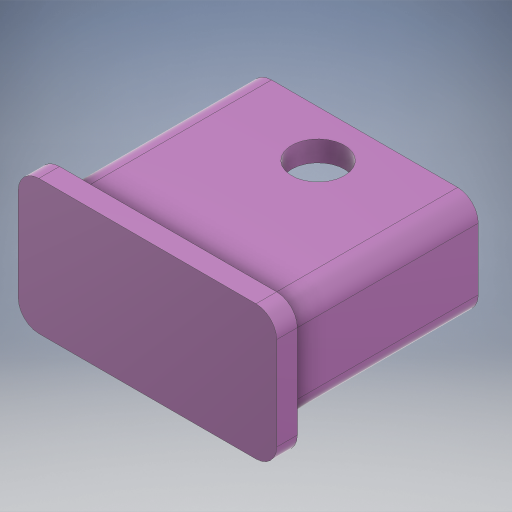
# Autodesk Inventor part: Короб подшипника
Saved by Autodesk Inventor 2023 (Build 270158000, 158)
## iProperties
Created: 2022-10-30
Part Number: Короб подшипника
Material: Типовые
Document SubType Name: Modeling
Designer: Admin
Density: 1 g/cm^3
Appearance: По умолчанию
Author: Admin
Autodesk Inventor part; units mm, degrees
ref_plane "YZ Plane" through (0, 0, 0) normal (1, 0, 0) x (0, 1, 0)
ref_plane "XZ Plane" through (0, 0, 0) normal (0, 1, 0) x (-1, 0, 0)
ref_plane "XY Plane" through (0, 0, 0) normal (0, 0, 1) x (1, 0, 0)
sketch "Эскиз1" plane through (0, 0, 0) normal (0, 0, 1) x (1, 0, 0)
  line L0 (-10.5, -6.5) -> (10.5, -6.5)
  line L1 (12.5, -4.5) -> (12.5, 4.5)
  line L2 (10.5, 6.5) -> (-10.5, 6.5)
  line L3 (-12.5, 4.5) -> (-12.5, -4.5)
  line L4 (-12.5, -6.5) -> (12.5, 6.5) construction
  line L5 (12.5, -6.5) -> (-12.5, 6.5) construction
  line L6 (-9, 5) -> (9, 5)
  line L7 (11, 3) -> (11, -3)
  line L8 (9, -5) -> (-9, -5)
  line L9 (-11, -3) -> (-11, 3)
  arc A0 (-10.5, 6.5) -> (-12.5, 4.5) centre (-10.5, 4.5) ccw
  arc A1 (12.5, 4.5) -> (10.5, 6.5) centre (10.5, 4.5) ccw
  arc A2 (10.5, -6.5) -> (12.5, -4.5) centre (10.5, -4.5) ccw
  arc A3 (-12.5, -4.5) -> (-10.5, -6.5) centre (-10.5, -4.5) ccw
  arc A4 (-9, 5) -> (-11, 3) centre (-9, 3) ccw
  arc A5 (11, 3) -> (9, 5) centre (9, 3) ccw
  arc A6 (9, -5) -> (11, -3) centre (9, -3) ccw
  arc A7 (-11, -3) -> (-9, -5) centre (-9, -3) ccw
  line L10 (-9, 3) -> (9, 3)
  line L11 (9, 3) -> (9, -3)
  line L12 (9, -3) -> (-9, -3)
  line L13 (-9, -3) -> (-9, 3)
  line L14 (-9, 3) -> (9, -3) construction
  line L15 (9, 3) -> (-9, -3) construction
  point P0 (0, 0)
  dimension "d0" = 25
  dimension "d1" = 13
  dimension "d2" = 1.5
  dimension "d3" = 2
  dimension "d6" = 18
  dimension "d7" = 6
  constraints: 32 end point, 16 point on circle, 16 tangent, 8 centre point, 8 point on line, 7 equal radius, 6 parallel, 4 midpoint, 3 perpendicular, 2 horizontal, 3 other
  measures "d0" distance of L4.end L5.end
  measures "d1" distance between parallel lines of L0 L2
  measures "d2" distance between parallel lines of L2 L6
  measures "d3" radius of A0
  measures "d6" distance of L11.end L12.end
  measures "d7" distance of L12.end L10.start
extrude "Выдавливание1" add sketch "Эскиз1" along normal blind 2 contours A3 L3 A0 L2 A1 L1 A2 L0 | L6 A5 L7 A6 L8 A7 L9 A4 | L10 L11 L12 L13
extrude "Выдавливание2" add sketch "Эскиз1" against normal blind 19 contours L6 A5 L7 A6 L8 A7 L9 A4
sketch "Эскиз2" plane through (-9, 5, 0) normal (0, 1, 0) x (1, 0, 0)
  circle A0 centre (9, 14.5) radius 2.55
  circle A1 centre (9, 14.5) radius 8
  line L0 (0, 19) -> (18, 19) projected
  line L1 (19.5, -2) -> (-1.5, -2) projected
  line L2 (5, 12.1906) -> (5, 16.8094) construction
  line L3 (5, 16.8094) -> (9, 19.1188) construction
  line L4 (9, 19.1188) -> (13, 16.8094) construction
  line L5 (13, 16.8094) -> (13, 12.1906) construction
  line L6 (13, 12.1906) -> (9, 9.8812) construction
  line L7 (9, 9.8812) -> (5, 12.1906) construction
  line L8 (18.1, 7) -> (0, 7) construction
  line L9 (19.5, 0) -> (-1.5, 0) construction
  point P0 (9, 0)
  point P1 (9, 22.5)
  point P2 (9, 19)
  point P3 (9, 17.05)
  dimension "d10" = 5.1
  dimension "d11" = 16
  dimension "d12" = 24.5
  dimension "d13" = 8
  dimension "d14" = 7
  constraints: 14 end point, 5 vertical alignment, 2 coincident, 1 horizontal, 1 midpoint, 1 vertical, 17 other
  measures "d12" distance from line of L1 point (9, 22.5)
  measures "d13" distance between parallel lines of L7 L4
  measures "d14" distance between parallel lines of L9 L8
extrude "Выдавливание3" cut sketch "Эскиз2" against normal through all contours A0
